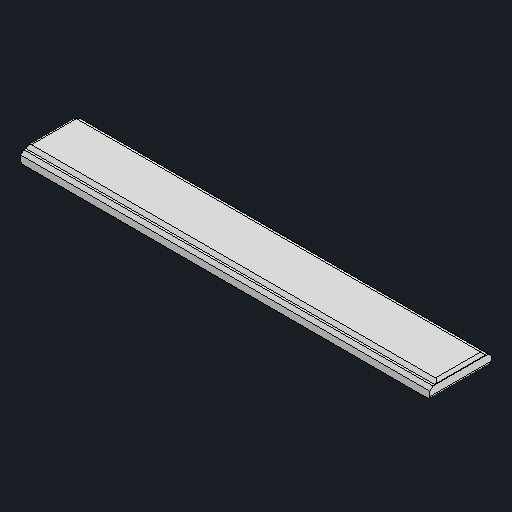
# Autodesk Inventor part: grip
Saved by Autodesk Inventor 2026 (Build 300175050, 175E)
## iProperties
Created: 2026-03-04
Part Number: grip
Material: Generic
Document SubType Name: Modeling
Designer: kuzmin
Density: 1 g/cm^3
Appearance: Default
Author: kuzmin
Autodesk Inventor part; units mm, degrees
ref_plane "YZ Plane" through (0, 0, 0) normal (1, 0, 0) x (0, 1, 0)
ref_plane "XZ Plane" through (0, 0, 0) normal (0, 1, 0) x (-1, 0, 0)
ref_plane "XY Plane" through (0, 0, 0) normal (0, 0, 1) x (1, 0, 0)
sketch "Sketch2" plane through (0, 0, 0) normal (0, 1, 0) x (-1, 0, 0)
  line L0 (40, 6) -> (-40, 6)
  line L1 (-40, 6) -> (-40, -6)
  line L2 (-40, -6) -> (40, -6)
  line L3 (40, -6) -> (40, 6)
  point P0 (0, 0)
  point P1 (0, -6)
  point P2 (40, 0)
  dimension "d1" = 80
  dimension "d2" = 12
  constraints: 8 end point, 2 midpoint, 2 parallel, 1 horizontal, 1 horizontal alignment, 1 perpendicular, 1 vertical alignment
  measures "d1" distance of L1.end L2.end
  measures "d2" distance of L2.end L0.start
extrude "Extrusion1" add sketch "Sketch2" along normal blind 2
sketch "Sketch3" plane through (0, 2, 0) normal (0, 1, 0) x (1, 0, 0)
  line L0 (-40, 6) -> (-40, -6) projected
  line L1 (-40, -5) -> (40, -5)
  line L2 (40, -5) -> (40, 5)
  line L3 (40, 5) -> (-40, 5)
  line L4 (-40, 5) -> (-40, -5)
  line L5 (40, -6) -> (40, 6) projected
  point P0 (0, 0)
  point P1 (-40, 0)
  dimension "d5" = 10
  constraints: 8 end point, 2 parallel, 2 point on line, 1 horizontal, 1 horizontal alignment, 1 midpoint, 1 perpendicular
  measures "d5" distance between parallel lines of L1 L3
extrude "Extrusion2" add sketch "Sketch3" along normal blind 0.6 separate body
chamfer "Chamfer1" distance 0.6 angle 45 2 edges at (0, 2.6, -5) (0, 2.6, 5)
chamfer "Chamfer2" distance 0.6 angle 45 2 edges at (0, 2, 6) (0, 2, -6)
fillet "Fillet1" radius 0.5 4 edges at (40, 0, 0) (-40, 0, 0) (40, 2.6, 0) (-40, 2.6, 0)
body "Solid1"
